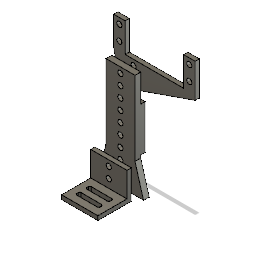
jaw servo holder (Autodesk Fusion 360 design; units mm, degrees)
Autodesk Fusion 360 part; units mm, degrees
sketch "Sketch1" plane through (0, 0, 0) normal (0, 0, 1) x (1, 0, 0)
  line L0 (-10, 71.5) -> (10, 71.5)
  line L1 (10, 71.5) -> (10, 0)
  line L2 (10, 0) -> (-10, 0)
  line L3 (-10, 0) -> (-10, 71.5)
  line L4 (0, 71.5) -> (0, 0) construction
  circle A0 centre (0, 75) radius 1.75
  circle A1 centre (0, 67.6667) radius 1.75
  circle A2 centre (0, 60.3333) radius 1.75
  circle A3 centre (0, 53) radius 1.75
  circle A4 centre (0, 45.6667) radius 1.75
  circle A5 centre (0, 38.3333) radius 1.75
  circle A6 centre (0, 31) radius 1.75
  circle A7 centre (0, 23.6667) radius 1.75
  circle A8 centre (0, 16.3333) radius 1.75
  circle A9 centre (0, 9) radius 1.75
  dimension "d1" = 20
  dimension "d2" = 71.5
  dimension "d3" = 3.5
  dimension "d17" = 0
  dimension "d18" = -66
  dimension "d52" = 9
  constraint horizontal L0
  constraint vertical L1
  constraint horizontal L2
  constraint vertical L3
  constraint midpoint L0 L4.start
  constraint midpoint L2 L4.end
  constraint coincident L4 A0.centre
  constraint coincident L4.end origin
  measures "d1" distance of L1 L3
  measures "d2" distance of L0 L2
  measures "d3" diameter of A0
  measures "d52" distance of L4.end A9.centre
sketch "Sketch3" plane through (0, 0, 0) normal (0, 0, 1) x (1, 0, 0) in component "base"
  line L0 (-12.5, 20.2418) -> (12.5, 20.2418)
  line L1 (12.5, 20.2418) -> (12.5, 0.2418)
  line L2 (12.5, 0.2418) -> (-12.5, 0.2418)
  line L3 (-12.5, 0.2418) -> (-12.5, 20.2418)
  line L4 (0, 20.2418) -> (0, 0) construction
  circle A0 centre (0, 16.3333) radius 1.75
  circle A1 centre (0, 9) radius 1.75
  dimension "d19" = 20
  dimension "d20" = 25
  constraint horizontal L0
  constraint vertical L1
  constraint horizontal L2
  constraint vertical L3
  constraint midpoint L0 L4.start
  constraint coincident L4.end origin
  constraint vertical L4
  measures "d19" distance of L0 L2
  measures "d20" distance of L1 L3
extrude "Extrude2" add sketch "Sketch3" along normal blind 3 makes body 1 in component "base"
sketch "Sketch4" plane through (0, 0, 3) normal (0, 0, 1) x (1, 0, 0) in component "base"
  circle A0 centre (0, 16.3333) radius 1.75
  circle A1 centre (0, 9) radius 1.75
  line L0 (-12.5, 0.2418) -> (12.5, 0.2418)
  line L1 (12.5, 0.2418) -> (12.5, 20.2418)
  line L2 (12.5, 20.2418) -> (-12.5, 20.2418)
  line L3 (-12.5, 20.2418) -> (-12.5, 0.2418)
  line L4 (-12.5, 0.2418) -> (12.5, 0.2418)
  line L5 (12.5, 0.2418) -> (12.5, 3.2418)
  line L6 (12.5, 3.2418) -> (-12.5, 3.2418)
  line L7 (-12.5, 3.2418) -> (-12.5, 0.2418)
  dimension "d23" = 3
  constraint horizontal L4
  constraint vertical L5
  constraint horizontal L6
  constraint vertical L7
  constraint coincident L1 L5.end
  constraint coincident L0.start L3.end
  measures "d23" distance of L4 L6
extrude "Extrude3" add sketch "Sketch4" along normal blind 20 contours L0 L1 L3 L4 L5 L6 L7 bodies 1 in component "base"
sketch "Sketch5" plane through (0, 3.2418, 0) normal (0, 1, 0) x (-1, 0, 0) in component "base"
  line L0 (-12.5, 3) -> (12.5, 3)
  line L1 (12.5, 3) -> (12.5, 23)
  line L2 (12.5, 23) -> (-12.5, 23)
  line L3 (-12.5, 23) -> (-12.5, 3)
  line L4 (7, 8) -> (-7, 8)
  line L5 (-8, 9) -> (-8, 10)
  line L6 (-7, 11) -> (7, 11)
  line L7 (8, 10) -> (8, 9)
  line L8 (0, 3) -> (0, 23) construction
  arc A0 (7, 8) -> (8, 9) centre (7, 9) ccw
  arc A1 (8, 10) -> (7, 11) centre (7, 10) ccw
  arc A2 (-8, 9) -> (-7, 8) centre (-7, 9) ccw
  arc A3 (-7, 11) -> (-8, 10) centre (-7, 10) ccw
  line L9 (0, 8) -> (0, 11) construction
  line L10 (12.5, 13) -> (-12.5, 13) construction
  line L11 (7, 18) -> (-7, 18)
  arc A4 (-7, 18) -> (-8, 17) centre (-7, 17) ccw
  line L12 (-8, 17) -> (-8, 16)
  arc A5 (-8, 16) -> (-7, 15) centre (-7, 16) ccw
  line L13 (-7, 15) -> (7, 15)
  arc A6 (7, 15) -> (8, 16) centre (7, 16) ccw
  line L14 (8, 16) -> (8, 17)
  arc A7 (8, 17) -> (7, 18) centre (7, 17) ccw
  dimension "d26" = 3
  dimension "d27" = 16
  dimension "d28" = 1
  dimension "d29" = 5
  constraint horizontal L4
  constraint vertical L5
  constraint horizontal L6
  constraint vertical L7
  constraint midpoint L0 L8.start
  constraint midpoint L2 L8.end
  constraint tangent L7 A0
  constraint tangent L4 A0
  constraint tangent L6 A1
  constraint tangent L7 A1
  constraint equal A0 A1
  constraint tangent L4 A2
  constraint tangent L5 A2
  constraint equal A0 A2
  constraint tangent L5 A3
  constraint tangent L6 A3
  constraint equal A0 A3
  constraint midpoint L4 L9.start
  constraint midpoint L6 L9.end
  constraint collinear L8 L9
  constraint midpoint L1 L10.start
  constraint midpoint L3 L10.end
  constraint symmetric L7.end L10 L14.end
  constraint symmetric L4.start L10 L11.start
  constraint symmetric A0 L10 A7
  constraint symmetric L6.end L10 L13.end
  constraint symmetric L7.start L10 A6.end
  constraint symmetric A1 L10 A6
  constraint symmetric L4.end L10 L11.end
  constraint symmetric L5.start L10 A4.end
  constraint symmetric A2 L10 A4
  constraint symmetric L5.end L10 L12.end
  constraint symmetric L6.start L10 A5.end
  constraint symmetric A3 L10 A5
  measures "d26" distance of L4 L6
  measures "d27" distance of L5 L7
  measures "d28" radius of A0
  measures "d29" distance of L0 L4
extrude "Extrude4" cut sketch "Sketch5" against normal up to surface (3 mm away) contours L4 L5 L6 L7 A0 A1 A2 A3 | L11 A4 L12 A5 L13 A6 L14 A7 bodies 1 in component "base"
sketch "Sketch1 (2)" plane through (0, 0, 0) normal (0, 0, 1) x (1, 0, 0) in component "standup"
extrude "Extrude1" add sketch "Sketch1" against normal blind 4 separate body contours L0 L1 L2 L3 makes body 2 in component "standup"
sketch "Sketch2" plane through (0, 0, -4) normal (0, 0, -1) x (-1, 0, 0) in component "standup"
  circle A0 centre (0, 23.6667) radius 1.75
  circle A1 centre (0, 38.3333) radius 1.75
  circle A2 centre (0, 45.6667) radius 1.75
  circle A3 centre (0, 9) radius 1.75
  circle A4 centre (0, 31) radius 1.75
  circle A5 centre (0, 67.6667) radius 1.75
  circle A6 centre (0, 53) radius 1.75
  circle A7 centre (0, 60.3333) radius 1.75
  circle A8 centre (0, 16.3333) radius 1.75
  line L0 (-10, 0) -> (10, 0)
  line L1 (10, 0) -> (10, 71.5)
  line L2 (10, 71.5) -> (-10, 71.5)
  line L3 (-10, 71.5) -> (-10, 0)
  line L4 (-10, 0) -> (-15.9079, 0)
  line L5 (-15.9079, 0) -> (-10, 20.298)
  line L6 (0, 71.5) -> (0, 0) construction
  line L7 (15.9079, 0) -> (10, 20.298)
  line L8 (10, 0) -> (15.9079, 0)
  constraint coincident L0.start L3.end
  constraint perpendicular L3 L4
  constraint coincident L3 L5.end
  constraint midpoint L2 L6.start
  constraint coincident L6.end origin
  constraint symmetric L0.start L6 L0.end
  constraint symmetric L4.end L6 L7.start
  constraint symmetric L5.end L6 L7.end
extrude "Extrude2'" add sketch "Sketch2" against normal blind 4 contours L3 L4 L5 | L1 L7 L8 bodies 2 in component "standup"
sketch "Sketch1 (3)" plane through (0, 0, -4) normal (0, 0, -1) x (-1, 0, 0) in component "servo holder"
  circle A0 centre (0, 23.6667) radius 1.75
  circle A1 centre (0, 38.3333) radius 1.75
  circle A2 centre (0, 45.6667) radius 1.75
  circle A3 centre (0, 9) radius 1.75
  circle A4 centre (0, 31) radius 1.75
  circle A5 centre (0, 67.6667) radius 1.75
  circle A6 centre (0, 53) radius 1.75
  circle A7 centre (0, 60.3333) radius 1.75
  circle A8 centre (0, 16.3333) radius 1.75
  line L0 (-15.9079, 0) -> (15.9079, 0)
  line L1 (15.9079, 0) -> (10, 20.298)
  line L2 (10, 20.298) -> (10, 71.5)
  line L3 (10, 71.5) -> (-10, 71.5)
  line L4 (-10, 71.5) -> (-10, 20.298)
  line L5 (-10, 20.298) -> (-15.9079, 0)
  line L6 (10, 71.5) -> (-10, 71.5)
  circle A9 centre (0, 75) radius 1.75
  circle A10 centre (0, 67.6667) radius 1.75
  line L7 (-10, 71.5) -> (-10, 20.298)
  line L8 (10, 20.298) -> (10, 71.5)
  line L9 (10, 71.5) -> (10, 53.5)
  line L10 (10, 53.5) -> (-42.2864, 53.5)
  line L11 (-42.2864, 53.5) -> (-42.2864, 80.2767)
  line L12 (-42.2864, 91.5) -> (-34.2864, 91.5)
  line L13 (-34.2864, 91.5) -> (-34.2864, 71.5)
  line L14 (-42.2864, 80.2767) -> (-42.2864, 91.5)
  line L15 (13.7136, 71.5) -> (13.7136, 91.5)
  line L16 (13.7136, 91.5) -> (5.7136, 91.5)
  line L17 (5.7136, 91.5) -> (5.7136, 71.5)
  line L18 (-34.2864, 71.5) -> (5.7136, 71.5)
  line L19 (13.7136, 71.5) -> (10, 71.5)
  line L20 (-38.2864, 91.5) -> (-38.2864, 74.3829) construction
  line L21 (9.7136, 91.5) -> (9.7136, 76.0852) construction
  circle A11 centre (-38.2864, 87.5) radius 1.75
  line L22 (-10, 71.5) -> (-10, 89.5208) construction
  circle A12 centre (9.7136, 87.5) radius 1.75
  line L23 (-42.2864, 68.1182) -> (-0.2995, 53.5)
  line L24 (-38.2864, 87.5) -> (18.7146, 87.5) construction
  line L25 (-38.2864, 77.5) -> (19.8378, 77.5) construction
  circle A13 centre (-38.2864, 77.5) radius 1.75
  circle A14 centre (9.7136, 77.5) radius 1.75
  line L26 (13.7136, 71.5) -> (10, 53.5)
  circle A15 centre (0, 60.3333) radius 1.75
  dimension "d36" = 8
  dimension "d37" = 8
  dimension "d39" = 18
  dimension "d41" = 40
  dimension "d42" = 20
  dimension "d43" = 3.5
  dimension "d46" = 48
  dimension "d48" = 4
  dimension "d49" = 10
  dimension "d50" = 3.5
  dimension "d51" = 3.5
  constraint horizontal L18
  constraint vertical L9
  constraint horizontal L10
  constraint vertical L11
  constraint coincident L2 L9.end
  constraint horizontal L12
  constraint vertical L13
  constraint vertical L14
  constraint vertical L15
  constraint horizontal L16
  constraint vertical L17
  constraint collinear L11 L14
  constraint collinear L12 L16
  constraint collinear L18 L19
  constraint coincident L2.end L3.start
  constraint midpoint L12 L20.start
  constraint perpendicular L12 L20
  constraint midpoint L16 L21.start
  constraint perpendicular L16 L21
  constraint coincident L20 A11.centre
  constraint coincident L3.end L4.start
  constraint perpendicular L18 L22
  constraint coincident L11 L23.start
  constraint coincident L10 L23.end
  constraint coincident A11.centre L24.start
  constraint perpendicular L15 L24
  constraint coincident A12.centre L24
  constraint coincident L20 L25.start
  constraint perpendicular L15 L25
  constraint coincident L25.start A13.centre
  constraint coincident L25 A14.centre
  constraint coincident L21 A14.centre
  measures "d36" distance of L12.start L12.end
  measures "d37" distance of L15 L17
  measures "d39" distance of L10 L18
  measures "d41" distance of L13 L17
  measures "d42" distance of L16 L19
  measures "d43" diameter of A11
  measures "d46" horizontal distance of A11.centre A12.centre
  measures "d48" distance of L20.start A11.centre
  measures "d49" distance of L24 L25
  measures "d50" diameter of A13
  measures "d51" diameter of A14
extrude "Extrude1'" add sketch "Sketch1 (3)" along normal blind 3 separate body contours A6 L10 L23 | A6 L2 L3 L4 L6 L7 L8 L9 L10 L18 L23 | L2 L8 L9 L19 L26 | L4 L7 L11 L12 L13 L14 L18 L23 | L3 L6 L15 L16 L17 L19 picked at (-0.6751, 54.1782) makes body 3 in component "servo holder"
move_body "Move1" bodies 3 to x (1, 0, 0) y (0, 1, 0) z (0, 0, 1) at (0, 0, -5) in component "servo holder"
move_body "Move1'" bodies 1 to x (1, 0, 0) y (0, 1, 0) z (0, 0, 1) at (0, 0, 5) in component "base"
sketch "Sketch3 (2)" plane through (0, 0, -4) normal (0, 0, -1) x (-1, 0, 0) in component "standup"
  circle A0 centre (0, 67.6667) radius 1.75
  circle A1 centre (0, 23.6667) radius 1.75
  circle A2 centre (0, 45.6667) radius 1.75
  circle A3 centre (0, 38.3333) radius 1.75
  circle A4 centre (0, 31) radius 1.75
  circle A5 centre (0, 9) radius 1.75
  circle A6 centre (0, 16.3333) radius 1.75
  circle A7 centre (0, 53) radius 1.75
  circle A8 centre (0, 60.3333) radius 1.75
  line L0 (-15.9079, 0) -> (15.9079, 0)
  line L1 (15.9079, 0) -> (10, 20.298)
  line L2 (10, 20.298) -> (10, 71.5)
  line L3 (10, 71.5) -> (-10, 71.5)
  line L4 (-10, 71.5) -> (-10, 20.298)
  line L5 (-10, 20.298) -> (-15.9079, 0)
  line L6 (-10, 52.4082) -> (-5, 52.4082)
  line L7 (-5, 52.4082) -> (-5, 22)
  line L8 (-5, 22) -> (-10, 22)
  line L9 (-10, 22) -> (-10, 52.4082)
  line L10 (10, 22) -> (5, 22)
  line L11 (5, 22) -> (5, 52.4082)
  line L12 (5, 52.4082) -> (10, 52.4082)
  line L13 (10, 52.4082) -> (10, 22)
  dimension "d53" = 5
  dimension "d54" = 5
  dimension "d55" = 22
  constraint horizontal L6
  constraint vertical L7
  constraint horizontal L8
  constraint vertical L9
  constraint coincident L4 L6.start
  constraint horizontal L10
  constraint vertical L11
  constraint horizontal L12
  constraint vertical L13
  constraint coincident L2 L12.end
  constraint collinear L8 L10
  constraint collinear L6 L12
  measures "d53" distance of L7 L9
  measures "d54" distance of L11 L13
  measures "d55" distance of L0 L8
extrude "Extrude3'" add sketch "Sketch3 (2)" along normal blind 3 contours L4 L6 L7 L8 L9 | L2 L10 L11 L12 L13 bodies 2 in component "standup"
component "base" placed x (1, 0, 0) y (0, 1, 0) z (0, 0, 1) at (0, 0, 0)
component "standup" placed x (1, 0, 0) y (0, 1, 0) z (0, 0, 1) at (0, 0, 0)
component "servo holder" placed x (1, 0, 0) y (0, 1, 0) z (0, 0, 1) at (0, 0, 0)
equation "d37 = d36"
equation "d54 = d53"
